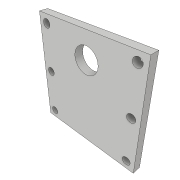
# Autodesk Inventor part: lift dc motor
Saved by Autodesk Inventor 2019 (Build 230136000, 136)
## iProperties
Created: 2019-10-07
Part Number: lift dc motor
Material: Generic
Document SubType Name: Modeling
Designer: Admin
Density: 1 g/cm^3
Appearance: Default
Author: Admin
Autodesk Inventor part; units mm, degrees
ref_plane "YZ Plane" through (0, 0, 0) normal (1, 0, 0) x (0, 1, 0)
ref_plane "XZ Plane" through (0, 0, 0) normal (0, 1, 0) x (-1, 0, 0)
ref_plane "XY Plane" through (0, 0, 0) normal (0, 0, 1) x (1, 0, 0)
sketch "Sketch1" plane through (0, 0, 0) normal (0, 0, 1) x (1, 0, 0)
  line L0 (0, 0) -> (130, 0)
  line L1 (130, 0) -> (130, 130)
  line L2 (130, 130) -> (0, 130)
  line L3 (0, 130) -> (0, 0)
  dimension "d0" = 130
  dimension "d1" = 130
  constraints: 8 end point, 2 parallel, 1 horizontal, 1 perpendicular
  measures "d0" distance of L2.end L1.end
  measures "d1" distance of L1.end L0.end
extrude "Extrusion1" add sketch "Sketch1" along normal blind 10
sketch "Sketch2" plane through (0, 0, 10) normal (0, 0, 1) x (1, 0, 0)
  line L0 (0, 130) -> (0, 0) projected
  line L1 (0, 130) -> (10, 130)
  line L2 (130, 130) -> (0, 130) projected
  line L3 (10, 130) -> (10, 0)
  line L4 (10, 0) -> (120, 0)
  line L5 (0, 0) -> (130, 0) projected
  line L6 (120, 0) -> (120, 130)
  line L7 (120, 130) -> (120, 120)
  line L8 (120, 120) -> (10, 120)
  line L9 (130, 0) -> (130, 130) projected
  line L10 (130, 0) -> (130, 10)
  line L11 (130, 10) -> (-3.175, 10)
  circle A0 centre (10, 10) radius 5
  circle A1 centre (120, 10) radius 5
  circle A2 centre (120, 120) radius 5
  circle A3 centre (10, 120) radius 5
  line L12 (0, 0) -> (0, 38.1)
  line L13 (0, 130) -> (0, 65)
  line L14 (0, 65) -> (130, 65)
  circle A4 centre (10, 65) radius 5
  circle A5 centre (120, 65) radius 5
  line L15 (0, 130) -> (65, 130)
  line L16 (65, 130) -> (65, 100)
  circle A6 centre (65, 100) radius 15
  dimension "d4" = 10
  dimension "d5" = 110
  dimension "d6" = 10
  dimension "d7" = 10
  dimension "d8" = 10
  dimension "d9" = 10
  dimension "d10" = 10
  dimension "d11" = 10
  dimension "d12" = 65
  dimension "d13" = 10
  dimension "d14" = 10
  dimension "d15" = 65
  dimension "d16" = 30
  dimension "d17" = 30
  constraints: 26 end point, 13 point on line, 7 centre point, 5 midpoint, 5 perpendicular, 3 coincident
  measures "d4" distance of L0.start L1.end
  measures "d5" distance of L3.end L4.end
  measures "d6" distance of L6.end L7.end
  measures "d7" distance of L5.end L10.end
  measures "d8" diameter of A0
  measures "d9" diameter of A1
  measures "d10" diameter of A2
  measures "d11" diameter of A3
  measures "d12" distance of L0.start L13.end
  measures "d13" diameter of A4
  measures "d14" diameter of A5
  measures "d15" distance of L0.start L15.end
  measures "d16" distance of L15.end L16.end
  measures "d17" diameter of A6
extrude "Extrusion2" cut sketch "Sketch2" against normal through all contours A4 L3 L14 | L14 L3 A4 | A3 L8 L3 | L3 A3 | L14 A4 L3 | L3 A4 L14 | A6 | L8 A3 L3 | A0 L3 L11 | L11 L3 A0 | A0 L11 L3 | A2 L6 | L6 L8 A2 | L8 L6 A2 | L11 A0 L3 | A5 L6 L14 | L14 L6 A5 | L14 A5 L6 | L6 A5 L14 | A1 L6 L11 | L11 L6 A1 | L6 L11 A1 | A1 L11 L6
body "Solid1"
